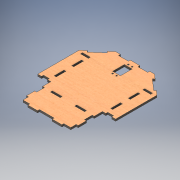
# Autodesk Inventor part: base
Saved by Autodesk Inventor 2019 (Build 230136000, 136)
## iProperties
Created: 2020-12-06
Part Number: base
Material: Дерево (береза)
Document SubType Name: Modeling
Designer: Professional
Density: 0.55 g/cm^3
Appearance: Береза — натуральный — полированный
Author: Professional
Autodesk Inventor part; units mm, degrees
ref_plane "YZ Plane" through (0, 0, 0) normal (1, 0, 0) x (0, 1, 0)
ref_plane "XZ Plane" through (0, 0, 0) normal (0, 1, 0) x (-1, 0, 0)
ref_plane "XY Plane" through (0, 0, 0) normal (0, 0, 1) x (1, 0, 0)
sketch "Эскиз1" plane through (0, 0, 0) normal (0, 1, 0) x (-1, 0, 0)
  line L0 (40, -185.2) -> (80, -150.2) construction
  line L1 (80, -150.2) -> (80, -65.2) construction
  line L2 (0, -185.2) -> (0, 0)
  line L3 (80, -65.2) -> (53, -65.2) construction
  line L4 (53, -65.2) -> (53, 0) construction
  line L5 (40, -185.2) -> (0, -185.2) construction
  line L6 (53, 0) -> (0, 0) construction
  line L7 (49, -15.2) -> (53, -15.2)
  line L8 (53, -15.2) -> (53, -32.2)
  line L9 (53, -32.2) -> (49, -32.2)
  line L10 (49, -32.2) -> (49, -48.2)
  line L11 (49, -48.2) -> (53, -48.2)
  line L12 (60, -65.2) -> (60, -69.2)
  line L13 (60, -69.2) -> (72, -69.2)
  line L14 (72, -69.2) -> (72, -65.2)
  line L15 (72, -65.2) -> (80, -65.2)
  line L16 (80, -65.2) -> (80, -150.2)
  line L17 (80, -150.2) -> (70.9691, -158.1021)
  line L18 (70.9691, -158.1021) -> (68.3351, -155.0917)
  line L19 (46.3969, -174.2876) -> (49.0309, -177.2979)
  line L20 (49.0309, -177.2979) -> (40, -185.2)
  line L21 (40, -185.2) -> (30, -185.2)
  line L22 (30, -185.2) -> (30, -181.2)
  line L23 (30, -181.2) -> (10, -181.2)
  line L24 (10, -181.2) -> (10, -185.2)
  line L25 (-40, -185.2) -> (-80, -150.2) construction
  line L26 (-80, -150.2) -> (-80, -65.2) construction
  line L27 (-80, -65.2) -> (-53, -65.2) construction
  line L28 (-53, -65.2) -> (-53, 0) construction
  line L29 (-40, -185.2) -> (0, -185.2) construction
  line L30 (-53, 0) -> (0, 0) construction
  line L31 (-49, -15.2) -> (-53, -15.2)
  line L32 (-53, -15.2) -> (-53, -32.2)
  line L33 (-53, -32.2) -> (-49, -32.2)
  line L34 (-49, -32.2) -> (-49, -48.2)
  line L35 (-49, -48.2) -> (-53, -48.2)
  line L36 (-60, -65.2) -> (-60, -69.2)
  line L37 (-60, -69.2) -> (-72, -69.2)
  line L38 (-72, -69.2) -> (-72, -65.2)
  line L39 (-72, -65.2) -> (-80, -65.2)
  line L40 (-80, -65.2) -> (-80, -150.2)
  line L41 (-40, -185.2) -> (-30, -185.2)
  line L42 (-30, -185.2) -> (-30, -181.2)
  line L43 (-30, -181.2) -> (-10, -181.2)
  line L44 (-10, -181.2) -> (-10, -185.2)
  line L45 (-10, -185.2) -> (10, -185.2)
  line L46 (68.3351, -155.0917) -> (46.3969, -174.2876)
  line L47 (-80, -150.2) -> (-70.9691, -158.1021)
  line L48 (-70.9691, -158.1021) -> (-68.3351, -155.0917)
  line L49 (-46.3969, -174.2876) -> (-49.0309, -177.2979)
  line L50 (-49.0309, -177.2979) -> (-40, -185.2)
  line L51 (-68.3351, -155.0917) -> (-46.3969, -174.2876)
  line L52 (60, -79.2) -> (56, -79.2)
  line L53 (56, -79.2) -> (56, -99.2)
  line L54 (56, -99.2) -> (60, -99.2)
  line L55 (60, -99.2) -> (60, -79.2)
  line L56 (60, -115.2) -> (56, -115.2)
  line L57 (56, -115.2) -> (56, -135.2)
  line L58 (56, -135.2) -> (60, -135.2)
  line L59 (60, -135.2) -> (60, -115.2)
  line L60 (72, -145.2) -> (56, -145.2)
  line L61 (56, -145.2) -> (56, -149.2)
  line L62 (56, -149.2) -> (72, -149.2)
  line L63 (72, -149.2) -> (72, -145.2)
  line L64 (-60, -79.2) -> (-56, -79.2)
  line L65 (-56, -79.2) -> (-56, -99.2)
  line L66 (-56, -99.2) -> (-60, -99.2)
  line L67 (-60, -99.2) -> (-60, -79.2)
  line L68 (-60, -115.2) -> (-56, -115.2)
  line L69 (-56, -115.2) -> (-56, -135.2)
  line L70 (-56, -135.2) -> (-60, -135.2)
  line L71 (-60, -135.2) -> (-60, -115.2)
  line L72 (-72, -145.2) -> (-56, -145.2)
  line L73 (-56, -145.2) -> (-56, -149.2)
  line L74 (-56, -149.2) -> (-72, -149.2)
  line L75 (-72, -149.2) -> (-72, -145.2)
  line L76 (40, -185.2) -> (40, -181.2) construction
  line L77 (40, -181.2) -> (30, -181.2) construction
  line L78 (53, -48.2) -> (53, -65.2)
  line L79 (60, -65.2) -> (53, -65.2)
  line L80 (-53, -48.2) -> (-53, -65.2)
  line L81 (-60, -65.2) -> (-53, -65.2)
  line L82 (49, -15.2) -> (49, -4)
  line L83 (49, -4) -> (35, -4)
  line L84 (35, -4) -> (35, 0)
  line L85 (35, 0) -> (15, 0)
  line L86 (15, 0) -> (15, -4)
  line L87 (15, -4) -> (0, -4)
  line L88 (-49, -4) -> (-35, -4)
  line L89 (-35, -4) -> (-35, 0)
  line L90 (-35, 0) -> (-15, 0)
  line L91 (-15, 0) -> (-15, -4)
  line L92 (-15, -4) -> (0, -4)
  line L93 (-49, -4) -> (-49, -15.2)
  line L94 (35, -46.4) -> (15, -46.4)
  line L95 (15, -46.4) -> (15, -50.4)
  line L96 (15, -50.4) -> (35, -50.4)
  line L97 (35, -50.4) -> (35, -46.4)
  line L98 (-15, -46.4) -> (-35, -46.4)
  line L99 (-35, -46.4) -> (-35, -50.4)
  line L100 (-35, -50.4) -> (-15, -50.4)
  line L101 (-15, -50.4) -> (-15, -46.4)
  line L102 (8, -147.2) -> (-8, -147.2)
  line L103 (-8, -147.2) -> (-8, -171.2)
  line L104 (-8, -171.2) -> (8, -171.2)
  line L105 (8, -171.2) -> (8, -147.2)
  line L106 (8, -147.2) -> (-8, -171.2) construction
  line L107 (-8, -147.2) -> (8, -171.2) construction
  point P0 (0, -159.2)
  dimension "d1" = 160
  dimension "d2" = 106
  dimension "d3" = 65.2
  dimension "d5" = 80
  dimension "d6" = 85
  dimension "d7" = 27
  dimension "d14" = 4
  dimension "d15" = 15.2
  dimension "d16" = 16
  dimension "d19" = 17
  dimension "d20" = 12
  dimension "d21" = 8
  dimension "d25" = 12
  dimension "d26" = 12
  dimension "d29" = 20
  dimension "d32" = 10
  dimension "d35" = 20
  dimension "d37" = 29.1507
  dimension "d38" = 20
  dimension "d39" = 20
  dimension "d40" = 16
  dimension "d41" = 10
  dimension "d42" = 16
  dimension "d44" = 10
  dimension "d45" = 8
  dimension "d46" = 1
  dimension "d47" = 17
  dimension "d48" = 35
  dimension "d50" = 20
  dimension "d51" = 30
  dimension "d52" = 14
  dimension "d53" = 20
  dimension "d54" = 30
  dimension "d55" = 46.4
  dimension "d56" = 24
  dimension "d57" = 16
  dimension "d58" = 10
  constraints: 217 end point, 41 symmetric about line, 27 point on line, 20 perpendicular, 13 parallel, 12 equal length, 11 horizontal, 8 vertical, 5 collinear, 2 midpoint, 1 vertical alignment, 2 other
  measures "d1" diameter of L1 L2
  measures "d2" diameter of L4 L2
  measures "d3" distance between parallel lines of L3 L6
  measures "d5" diameter of L0.start L2
  measures "d6" distance of L0.end L1.end
  measures "d7" distance between parallel lines of L1 L4
  measures "d14" distance of L10.end L11.end
  measures "d15" distance between parallel lines of L6 L7
  measures "d16" distance between parallel lines of L11 L9
  measures "d19" distance between parallel lines of L7 L9
  measures "d20" distance between parallel lines of L14 L12
  measures "d21" distance between parallel lines of L1 L14
  measures "d25" distance from line of L18 L0.end
  measures "d26" distance from line of L19 L0.start
  measures "d29" distance between parallel lines of L22 L24
  measures "d32" distance from line of L0.start L22
  measures "d35" distance between parallel lines of L44 L24
  measures "d37" distance between parallel lines of L19 L18
  measures "d38" distance of L58.end L56.start
  measures "d39" distance between parallel lines of L1 L55
  measures "d40" distance between parallel lines of L54 L56
  measures "d41" distance between parallel lines of L13 L52
  measures "d42" distance of L60.start L60.end
  measures "d44" distance between parallel lines of L58 L60
  measures "d45" distance between parallel lines of L1 L63
  measures "d46" distance from line of L0.end L62
  measures "d47" distance between parallel lines of L11 L3
  measures "d48" distance from line of L21 L0.end
  measures "d50" distance between parallel lines of L86 L84
  measures "d51" diameter of L86 L2
  measures "d52" distance between parallel lines of L82 L84
  measures "d53" distance of L95.end L96.end
  measures "d54" distance between parallel lines of L101 L95
  measures "d55" distance between parallel lines of L94 L85
  measures "d56" distance between parallel lines of L102 L104
  measures "d57" distance between parallel lines of L103 L105
  measures "d58" distance between parallel lines of L23 L104
extrude "Выдавливание1" add sketch "Эскиз1" along normal blind 4 contours L45 L44 L43 L42 L41 L50 L49 L51 L48 L47 L40 L39 L38 L37 L36 L81 L80 L35 L34 L33 L32 L31 L93 L88 L89 L90 L91 L92 L2 L102 L103 L104 | L2 L104 L105 L102 L87 L86 L85 L84 L83 L82 L7 L8 L9 L10 L11 L78 L79 L12 L13 L14 L15 L16 L17 L18 L46 L19 L20 L21 L22 L23 L24 L45
sketch "Эскиз3" plane through (0, 4, 0) normal (0, 1, 0) x (1, 0, 0)
  line L0 (-8, 147.2) -> (-8, 171.2) projected
  line L1 (-8, 159.2) -> (8, 159.2)
  line L2 (8, 171.2) -> (8, 147.2) projected
  line L3 (-8, 171.2) -> (8, 171.2) projected
  line L4 (0, 171.2) -> (0, 158.8523)
  point P0 (0, 0)
  point P1 (-4, 143.2)
  point P2 (4, 143.2)
  point P3 (-4, 175.2)
  point P4 (4, 175.2)
  dimension "d66" = 8
  dimension "d67" = 32
  constraints: 4 end point, 3 midpoint, 3 symmetric about line, 1 horizontal alignment, 1 vertical
  measures "d66" distance of point (-4, 175.2) point (4, 175.2)
  measures "d67" distance of point (4, 143.2) point (4, 175.2)
hole "Отверстие1" at (-4, 4, -143.2) at (4, 4, -143.2) at (-4, 4, -175.2) at (4, 4, -175.2) direction (0, -1, 0) diameter 2.8 end through all
